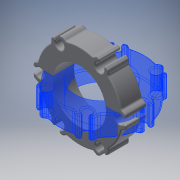
# Autodesk Inventor part: New Spacer
Saved by Autodesk Inventor 2017 (Build 210142000, 142)
## iProperties
Created: 2019-02-09
Part Number: New Spacer
Material: Generic
Document SubType Name: Modeling
Designer: S346795925
Density: 1 g/cm^3
Appearance: Default
Author: S346795925
Autodesk Inventor part; units mm, degrees
ref_plane "YZ Plane" through (0, 0, 0) normal (1, 0, 0) x (0, 1, 0)
ref_plane "XZ Plane" through (0, 0, 0) normal (0, 1, 0) x (-1, 0, 0)
ref_plane "XY Plane" through (0, 0, 0) normal (0, 0, 1) x (1, 0, 0)
sketch "Sketch1" plane through (0, 0, 0) normal (0, 0, 1) x (1, 0, 0)
  arc A0 (-16.7237, 21.3145) -> (-16.6929, 19.7418) centre (-11.9062, 20.6222) ccw construction
  arc A1 (-17.2068, 18.1665) -> (-16.6929, 19.7418) centre (-18.4013, 19.4276) ccw construction
  arc A2 (-17.2068, 18.1665) -> (-24.336, 5.8183) centre (0, 0) ccw construction
  arc A3 (-25.4434, 4.5856) -> (-24.336, 5.8183) centre (-26.0254, 6.2222) ccw construction
  arc A4 (-25.4434, 4.5856) -> (-26.8208, 3.8259) centre (-23.8125, 0) ccw construction
  arc A5 (-26.8208, 3.8259) -> (-27.1216, 3.2914) centre (-26.3245, 3.1947) ccw construction
  arc A6 (-27.1216, 3.2914) -> (-27.2147, 2.4031) centre (0, 0) ccw construction
  arc A7 (-27.2147, 2.4031) -> (-26.8956, 2.0545) centre (-26.8956, 2.3749) ccw construction
  line L0 (-26.8956, 2.0545) -> (-26.215, 2.0545) construction
  arc A8 (-26.215, 2.0545) -> (-25.9872, 2.1497) centre (-26.215, 2.3749) ccw construction
  arc A9 (-25.9872, -2.1497) -> (-25.9872, 2.1497) centre (-23.8125, 0) ccw construction
  arc A10 (-25.9872, -2.1497) -> (-26.215, -2.0545) centre (-26.215, -2.3749) ccw construction
  line L1 (-26.215, -2.0545) -> (-26.8956, -2.0545) construction
  arc A11 (-26.8956, -2.0545) -> (-27.2147, -2.4031) centre (-26.8956, -2.3749) ccw construction
  arc A12 (-27.2147, -2.4031) -> (-27.1216, -3.2914) centre (0, 0) ccw construction
  arc A13 (-27.1216, -3.2914) -> (-26.8208, -3.8259) centre (-26.3245, -3.1947) ccw construction
  arc A14 (-26.8208, -3.8259) -> (-24.5552, -4.81) centre (-23.8125, 0) ccw construction
  arc A15 (-24.5552, -4.81) -> (-17.2068, -18.1665) centre (0, 0) ccw construction
  arc A16 (-16.6929, -19.7418) -> (-17.2068, -18.1665) centre (-18.4013, -19.4276) ccw construction
  arc A17 (-16.6929, -19.7418) -> (-16.7237, -21.3145) centre (-11.9062, -20.6222) ccw construction
  arc A18 (-16.7237, -21.3145) -> (-16.4113, -21.8422) centre (-15.9289, -21.2003) ccw construction
  arc A19 (-16.4113, -21.8422) -> (-15.6885, -22.3671) centre (0, 0) ccw construction
  arc A20 (-15.6885, -22.3671) -> (-15.2271, -22.265) centre (-15.5045, -22.1048) ccw construction
  line L2 (-15.2271, -22.265) -> (-14.8868, -21.6756) construction
  arc A21 (-14.8868, -21.6756) -> (-14.8553, -21.4307) centre (-15.1642, -21.5154) ccw construction
  arc A22 (-11.1319, -23.5804) -> (-14.8553, -21.4307) centre (-11.9062, -20.6222) ccw construction
  arc A23 (-11.1319, -23.5804) -> (-11.3282, -23.7301) centre (-11.0508, -23.8903) ccw construction
  line L3 (-11.3282, -23.7301) -> (-11.6685, -24.3195) construction
  arc A24 (-11.6685, -24.3195) -> (-11.5262, -24.7701) centre (-11.3911, -24.4797) ccw construction
  arc A25 (-11.5262, -24.7701) -> (-10.7103, -25.1337) centre (0, 0) ccw construction
  arc A26 (-10.7103, -25.1337) -> (-10.097, -25.1404) centre (-10.3955, -24.395) ccw construction
  arc A27 (-10.097, -25.1404) -> (-8.7504, -24.3274) centre (-11.9062, -20.6222) ccw construction
  arc A28 (-7.1292, -23.9847) -> (-8.7504, -24.3274) centre (-7.6241, -25.6498) ccw construction
  arc A29 (-7.1292, -23.9847) -> (7.1292, -23.9847) centre (0, 0) ccw construction
  arc A30 (8.7504, -24.3274) -> (7.1292, -23.9847) centre (7.6241, -25.6498) ccw construction
  arc A31 (8.7504, -24.3274) -> (10.097, -25.1404) centre (11.9063, -20.6222) ccw construction
  arc A32 (10.097, -25.1404) -> (10.7103, -25.1337) centre (10.3955, -24.395) ccw construction
  arc A33 (10.7103, -25.1337) -> (11.5262, -24.7701) centre (0, 0) ccw construction
  arc A34 (11.5262, -24.7701) -> (11.6685, -24.3195) centre (11.3911, -24.4797) ccw construction
  line L4 (11.6685, -24.3195) -> (11.3282, -23.7301) construction
  arc A35 (11.3282, -23.7301) -> (11.1319, -23.5804) centre (11.0508, -23.8903) ccw construction
  arc A36 (14.8553, -21.4307) -> (11.1319, -23.5804) centre (11.9063, -20.6222) ccw construction
  arc A37 (14.8553, -21.4307) -> (14.8868, -21.6756) centre (15.1642, -21.5154) ccw construction
  line L5 (14.8868, -21.6756) -> (15.2271, -22.265) construction
  arc A38 (15.2271, -22.265) -> (15.6885, -22.3671) centre (15.5045, -22.1048) ccw construction
  arc A39 (15.6885, -22.3671) -> (16.4113, -21.8422) centre (0, 0) ccw construction
  arc A40 (16.4113, -21.8422) -> (16.7237, -21.3145) centre (15.9289, -21.2003) ccw construction
  arc A41 (16.7237, -21.3145) -> (16.6929, -19.7418) centre (11.9063, -20.6222) ccw construction
  arc A42 (17.2068, -18.1665) -> (16.6929, -19.7418) centre (18.4013, -19.4276) ccw construction
  arc A43 (17.2068, -18.1665) -> (24.336, -5.8183) centre (0, 0) ccw construction
  arc A44 (25.4434, -4.5856) -> (24.336, -5.8183) centre (26.0254, -6.2222) ccw construction
  arc A45 (25.4434, -4.5856) -> (26.8208, -3.8259) centre (23.8125, 0) ccw construction
  arc A46 (26.8208, -3.8259) -> (27.1216, -3.2914) centre (26.3245, -3.1947) ccw construction
  arc A47 (27.1216, -3.2914) -> (27.2147, -2.4031) centre (0, 0) ccw construction
  arc A48 (27.2147, -2.4031) -> (26.8956, -2.0545) centre (26.8956, -2.3749) ccw construction
  line L6 (26.8956, -2.0545) -> (26.215, -2.0545) construction
  arc A49 (26.215, -2.0545) -> (25.9872, -2.1497) centre (26.215, -2.3749) ccw construction
  arc A50 (25.9872, 2.1497) -> (25.9872, -2.1497) centre (23.8125, 0) ccw construction
  arc A51 (25.9872, 2.1497) -> (26.215, 2.0545) centre (26.215, 2.3749) ccw construction
  line L7 (26.215, 2.0545) -> (26.8956, 2.0545) construction
  arc A52 (26.8956, 2.0545) -> (27.2147, 2.4031) centre (26.8956, 2.3749) ccw construction
  arc A53 (27.2147, 2.4031) -> (27.1216, 3.2914) centre (0, 0) ccw construction
  arc A54 (27.1216, 3.2914) -> (26.8208, 3.8259) centre (26.3245, 3.1947) ccw construction
  arc A55 (26.8208, 3.8259) -> (25.4434, 4.5856) centre (23.8125, 0) ccw construction
  arc A56 (24.336, 5.8183) -> (25.4434, 4.5856) centre (26.0254, 6.2222) ccw construction
  arc A57 (24.336, 5.8183) -> (17.2068, 18.1665) centre (0, 0) ccw construction
  arc A58 (16.6929, 19.7418) -> (17.2068, 18.1665) centre (18.4013, 19.4276) ccw construction
  arc A59 (16.6929, 19.7418) -> (16.7237, 21.3145) centre (11.9063, 20.6222) ccw construction
  arc A60 (16.7237, 21.3145) -> (16.4113, 21.8422) centre (15.9289, 21.2003) ccw construction
  arc A61 (16.4113, 21.8422) -> (15.6885, 22.3671) centre (0, 0) ccw construction
  arc A62 (15.6885, 22.3671) -> (15.2271, 22.265) centre (15.5045, 22.1048) ccw construction
  line L8 (15.2271, 22.265) -> (14.8868, 21.6756) construction
  arc A63 (14.8868, 21.6756) -> (14.8553, 21.4307) centre (15.1642, 21.5154) ccw construction
  arc A64 (11.1319, 23.5804) -> (14.8553, 21.4307) centre (11.9063, 20.6222) ccw construction
  arc A65 (11.1319, 23.5804) -> (11.3282, 23.7301) centre (11.0508, 23.8903) ccw construction
  line L9 (11.3282, 23.7301) -> (11.6685, 24.3195) construction
  arc A66 (11.6685, 24.3195) -> (11.5262, 24.7701) centre (11.3911, 24.4797) ccw construction
  arc A67 (11.5262, 24.7701) -> (10.7103, 25.1337) centre (0, 0) ccw construction
  arc A68 (10.7103, 25.1337) -> (10.097, 25.1404) centre (10.3955, 24.395) ccw construction
  arc A69 (10.097, 25.1404) -> (8.7504, 24.3274) centre (11.9063, 20.6222) ccw construction
  arc A70 (7.1292, 23.9847) -> (8.7504, 24.3274) centre (7.6241, 25.6498) ccw construction
  arc A71 (7.1292, 23.9847) -> (-7.1292, 23.9847) centre (0, 0) ccw construction
  arc A72 (-8.7504, 24.3274) -> (-7.1292, 23.9847) centre (-7.6241, 25.6498) ccw construction
  arc A73 (-8.7504, 24.3274) -> (-10.097, 25.1404) centre (-11.9062, 20.6222) ccw construction
  arc A74 (-10.097, 25.1404) -> (-10.7103, 25.1337) centre (-10.3955, 24.395) ccw construction
  arc A75 (-10.7103, 25.1337) -> (-11.5262, 24.7701) centre (0, 0) ccw construction
  arc A76 (-11.5262, 24.7701) -> (-11.6685, 24.3195) centre (-11.3911, 24.4797) ccw construction
  line L10 (-11.6685, 24.3195) -> (-11.3282, 23.7301) construction
  arc A77 (-11.3282, 23.7301) -> (-11.1319, 23.5804) centre (-11.0508, 23.8903) ccw construction
  arc A78 (-14.8553, 21.4307) -> (-11.1319, 23.5804) centre (-11.9062, 20.6222) ccw construction
  arc A79 (-14.8553, 21.4307) -> (-14.8868, 21.6756) centre (-15.1642, 21.5154) ccw construction
  line L11 (-14.8868, 21.6756) -> (-15.2271, 22.265) construction
  arc A80 (-15.2271, 22.265) -> (-15.6885, 22.3671) centre (-15.5045, 22.1048) ccw construction
  arc A81 (-15.6885, 22.3671) -> (-16.4113, 21.8422) centre (0, 0) ccw construction
  arc A82 (-16.4113, 21.8422) -> (-16.7237, 21.3145) centre (-15.9289, 21.2003) ccw construction
  circle A83 centre (0, 0) radius 16.138 construction
  arc A84 (-24.9427, -5.2035) -> (-17.5216, -18.4989) centre (0, 0) ccw construction
  circle A85 centre (0, 0) radius 15.8842 projected
  arc A86 (-24.9427, -5.2035) -> (-17.5216, -18.4989) centre (0, 0) ccw
  arc A87 (-27.1038, -4.1858) -> (-24.9427, -5.2035) centre (-23.8125, 0) ccw
  arc A88 (-27.5761, -3.3466) -> (-27.1038, -4.1858) centre (-26.3245, -3.1947) ccw
  arc A89 (-27.6708, -2.4434) -> (-27.5761, -3.3466) centre (0, 0) ccw
  arc A90 (-26.8956, -1.5967) -> (-27.6708, -2.4434) centre (-26.8956, -2.3749) ccw
  line L12 (-26.8956, -1.5967) -> (-26.215, -1.5967)
  arc A91 (-25.6616, -1.8278) -> (-26.215, -1.5967) centre (-26.215, -2.3749) ccw
  arc A92 (-25.6616, -1.8278) -> (-25.6616, 1.8278) centre (-23.8125, 0) ccw
  arc A93 (-26.215, 1.5967) -> (-25.6616, 1.8278) centre (-26.215, 2.3749) ccw
  line L13 (-26.215, 1.5967) -> (-26.8956, 1.5967)
  arc A94 (-27.6708, 2.4434) -> (-26.8956, 1.5967) centre (-26.8956, 2.3749) ccw
  arc A95 (-27.5761, 3.3466) -> (-27.6708, 2.4434) centre (0, 0) ccw
  arc A96 (-27.1038, 4.1858) -> (-27.5761, 3.3466) centre (-26.3245, 3.1947) ccw
  arc A97 (-25.5968, 5.017) -> (-27.1038, 4.1858) centre (-23.8125, 0) ccw
  arc A98 (-25.5968, 5.017) -> (-24.7813, 5.9248) centre (-26.0254, 6.2222) ccw
  arc A99 (-17.5216, 18.4989) -> (-24.7813, 5.9248) centre (0, 0) ccw
  arc A100 (-17.5216, 18.4989) -> (-17.1432, 19.659) centre (-18.4013, 19.4276) ccw
  arc A101 (-17.1769, 21.3796) -> (-17.1432, 19.659) centre (-11.9062, 20.6222) ccw
  arc A102 (-16.6863, 22.2083) -> (-17.1769, 21.3796) centre (-15.9289, 21.2003) ccw
  arc A103 (-15.9514, 22.7419) -> (-16.6863, 22.2083) centre (0, 0) ccw
  arc A104 (-14.8305, 22.4939) -> (-15.9514, 22.7419) centre (-15.5045, 22.1048) ccw
  line L14 (-14.8305, 22.4939) -> (-14.4903, 21.9045)
  arc A105 (-14.4137, 21.3097) -> (-14.4903, 21.9045) centre (-15.1642, 21.5154) ccw
  arc A106 (-14.4137, 21.3097) -> (-11.2479, 23.1375) centre (-11.9062, 20.6222) ccw
  arc A107 (-11.7247, 23.5012) -> (-11.2479, 23.1375) centre (-11.0508, 23.8903) ccw
  line L15 (-11.7247, 23.5012) -> (-12.065, 24.0906)
  arc A108 (-11.7194, 25.1853) -> (-12.065, 24.0906) centre (-11.3911, 24.4797) ccw
  arc A109 (-10.8898, 25.5549) -> (-11.7194, 25.1853) centre (0, 0) ccw
  arc A110 (-9.9268, 25.5655) -> (-10.8898, 25.5549) centre (-10.3955, 24.395) ccw
  arc A111 (-8.4536, 24.676) -> (-9.9268, 25.5655) centre (-11.9062, 20.6222) ccw
  arc A112 (-8.4536, 24.676) -> (-7.2597, 24.4236) centre (-7.6241, 25.6498) ccw
  arc A113 (7.2597, 24.4236) -> (-7.2597, 24.4236) centre (0, 0) ccw
  arc A114 (7.2597, 24.4236) -> (8.4536, 24.676) centre (7.6241, 25.6498) ccw
  arc A115 (9.9268, 25.5655) -> (8.4536, 24.676) centre (11.9063, 20.6222) ccw
  arc A116 (10.8898, 25.5549) -> (9.9268, 25.5655) centre (10.3955, 24.395) ccw
  arc A117 (11.7194, 25.1853) -> (10.8898, 25.5549) centre (0, 0) ccw
  arc A118 (12.065, 24.0906) -> (11.7194, 25.1853) centre (11.3911, 24.4797) ccw
  line L16 (12.065, 24.0906) -> (11.7247, 23.5012)
  arc A119 (11.2479, 23.1375) -> (11.7247, 23.5012) centre (11.0508, 23.8903) ccw
  arc A120 (11.2479, 23.1375) -> (14.4137, 21.3097) centre (11.9063, 20.6222) ccw
  arc A121 (14.4903, 21.9045) -> (14.4137, 21.3097) centre (15.1642, 21.5154) ccw
  line L17 (14.4903, 21.9045) -> (14.8305, 22.4939)
  arc A122 (15.9514, 22.7419) -> (14.8305, 22.4939) centre (15.5045, 22.1048) ccw
  arc A123 (16.6863, 22.2083) -> (15.9514, 22.7419) centre (0, 0) ccw
  arc A124 (17.1769, 21.3796) -> (16.6863, 22.2083) centre (15.9289, 21.2003) ccw
  arc A125 (17.1432, 19.659) -> (17.1769, 21.3796) centre (11.9063, 20.6222) ccw
  arc A126 (17.1432, 19.659) -> (17.5216, 18.4989) centre (18.4013, 19.4276) ccw
  arc A127 (24.7813, 5.9248) -> (17.5216, 18.4989) centre (0, 0) ccw
  arc A128 (24.7813, 5.9248) -> (25.5968, 5.017) centre (26.0254, 6.2222) ccw
  arc A129 (27.1038, 4.1858) -> (25.5968, 5.017) centre (23.8125, 0) ccw
  arc A130 (27.5761, 3.3466) -> (27.1038, 4.1858) centre (26.3245, 3.1947) ccw
  arc A131 (27.6708, 2.4434) -> (27.5761, 3.3466) centre (0, 0) ccw
  arc A132 (26.8956, 1.5967) -> (27.6708, 2.4434) centre (26.8956, 2.3749) ccw
  line L18 (26.8956, 1.5967) -> (26.215, 1.5967)
  arc A133 (25.6616, 1.8278) -> (26.215, 1.5967) centre (26.215, 2.3749) ccw
  arc A134 (25.6616, 1.8278) -> (25.6616, -1.8278) centre (23.8125, 0) ccw
  arc A135 (26.215, -1.5967) -> (25.6616, -1.8278) centre (26.215, -2.3749) ccw
  line L19 (26.215, -1.5967) -> (26.8956, -1.5967)
  arc A136 (27.6708, -2.4434) -> (26.8956, -1.5967) centre (26.8956, -2.3749) ccw
  arc A137 (27.5761, -3.3466) -> (27.6708, -2.4434) centre (0, 0) ccw
  arc A138 (27.1038, -4.1858) -> (27.5761, -3.3466) centre (26.3245, -3.1947) ccw
  arc A139 (25.5968, -5.017) -> (27.1038, -4.1858) centre (23.8125, 0) ccw
  arc A140 (25.5968, -5.017) -> (24.7813, -5.9248) centre (26.0254, -6.2222) ccw
  arc A141 (17.5216, -18.4989) -> (24.7813, -5.9248) centre (0, 0) ccw
  arc A142 (17.5216, -18.4989) -> (17.1432, -19.659) centre (18.4013, -19.4276) ccw
  arc A143 (17.1769, -21.3796) -> (17.1432, -19.659) centre (11.9063, -20.6222) ccw
  arc A144 (16.6863, -22.2083) -> (17.1769, -21.3796) centre (15.9289, -21.2003) ccw
  arc A145 (15.9514, -22.7419) -> (16.6863, -22.2083) centre (0, 0) ccw
  arc A146 (14.8305, -22.4939) -> (15.9514, -22.7419) centre (15.5045, -22.1048) ccw
  line L20 (14.8305, -22.4939) -> (14.4903, -21.9045)
  arc A147 (14.4137, -21.3097) -> (14.4903, -21.9045) centre (15.1642, -21.5154) ccw
  arc A148 (14.4137, -21.3097) -> (11.2479, -23.1375) centre (11.9063, -20.6222) ccw
  arc A149 (11.7247, -23.5012) -> (11.2479, -23.1375) centre (11.0508, -23.8903) ccw
  line L21 (11.7247, -23.5012) -> (12.065, -24.0906)
  arc A150 (11.7194, -25.1853) -> (12.065, -24.0906) centre (11.3911, -24.4797) ccw
  arc A151 (10.8898, -25.5549) -> (11.7194, -25.1853) centre (0, 0) ccw
  arc A152 (9.9268, -25.5655) -> (10.8898, -25.5549) centre (10.3955, -24.395) ccw
  arc A153 (8.4536, -24.676) -> (9.9268, -25.5655) centre (11.9063, -20.6222) ccw
  arc A154 (8.4536, -24.676) -> (7.2597, -24.4236) centre (7.6241, -25.6498) ccw
  arc A155 (-7.2597, -24.4236) -> (7.2597, -24.4236) centre (0, 0) ccw
  arc A156 (-7.2597, -24.4236) -> (-8.4536, -24.676) centre (-7.6241, -25.6498) ccw
  arc A157 (-9.9268, -25.5655) -> (-8.4536, -24.676) centre (-11.9062, -20.6222) ccw
  arc A158 (-10.8898, -25.5549) -> (-9.9268, -25.5655) centre (-10.3955, -24.395) ccw
  arc A159 (-11.7194, -25.1853) -> (-10.8898, -25.5549) centre (0, 0) ccw
  arc A160 (-12.065, -24.0906) -> (-11.7194, -25.1853) centre (-11.3911, -24.4797) ccw
  line L22 (-12.065, -24.0906) -> (-11.7247, -23.5012)
  arc A161 (-11.2479, -23.1375) -> (-11.7247, -23.5012) centre (-11.0508, -23.8903) ccw
  arc A162 (-11.2479, -23.1375) -> (-14.4137, -21.3097) centre (-11.9062, -20.6222) ccw
  arc A163 (-14.4903, -21.9045) -> (-14.4137, -21.3097) centre (-15.1642, -21.5154) ccw
  line L23 (-14.4903, -21.9045) -> (-14.8305, -22.4939)
  arc A164 (-15.9514, -22.7419) -> (-14.8305, -22.4939) centre (-15.5045, -22.1048) ccw
  arc A165 (-16.6863, -22.2083) -> (-15.9514, -22.7419) centre (0, 0) ccw
  arc A166 (-17.1769, -21.3796) -> (-16.6863, -22.2083) centre (-15.9289, -21.2003) ccw
  arc A167 (-17.1432, -19.659) -> (-17.1769, -21.3796) centre (-11.9062, -20.6222) ccw
  arc A168 (-17.1432, -19.659) -> (-17.5216, -18.4989) centre (-18.4013, -19.4276) ccw
  constraints: 166 point on circle, 83 centre point, 24 end point, 94 other
extrude "Extrusion1" add sketch "Sketch1" along normal blind 12.7
fillet "Fillet1" radius 0.762 190 edges at (17.1852, 19.0309, 12.7) (17.23, 20.5179, 12.7) (17.0138, 21.8426, 12.7) (16.321, 22.4781, 12.7) (15.3364, 22.8646, 12.7) (14.6604, 22.1992, 12.7) (14.3924, 21.6148, 12.7) (10.6063, 18.3706, 12.7) (11.5227, 23.2715, 12.7) (11.8949, 23.7959, 12.7) (12.1332, 24.714, 12.7) (11.3061, 25.3735, 12.7) (10.4094, 25.6557, 12.7) (9.154, 25.1806, 12.7) (7.8886, 24.3983, 12.7) (0, 25.4797, 12.7) (-7.8886, 24.3983, 12.7) (-9.154, 25.1806, 12.7) (-10.4094, 25.6557, 12.7) (-11.3061, 25.3735, 12.7) (-12.1332, 24.714, 12.7) (-11.8949, 23.7959, 12.7) (-11.5227, 23.2715, 12.7) (-10.6063, 18.3706, 12.7) (-14.3924, 21.6148, 12.7) (-14.6604, 22.1992, 12.7) (-15.3364, 22.8646, 12.7) (-16.321, 22.4781, 12.7) (-17.0138, 21.8426, 12.7) (-17.23, 20.5179, 12.7) (-17.1852, 19.0309, 12.7) (-22.0661, 12.7399, 12.7) (-25.0738, 5.3674, 12.7) (-26.3841, 4.6627, 12.7) (-27.4232, 3.8131, 12.7) (-27.6271, 2.8954, 12.7) (-27.4695, 1.8494, 12.7) (-26.5553, 1.5967, 12.7) (-25.9151, 1.6568, 12.7) (-21.2125, 0, 12.7) (-25.9151, -1.6568, 12.7) (-26.5553, -1.5967, 12.7) (-27.4695, -1.8494, 12.7) (-27.6271, -2.8954, 12.7) (-27.4232, -3.8131, 12.7) (-26.081, -4.8174, 12.7) (25.0738, 5.3674, 12.7) (26.3841, 4.6627, 12.7) (27.4232, 3.8131, 12.7) (27.6271, 2.8954, 12.7) (27.4695, 1.8494, 12.7) (26.5553, 1.5967, 12.7) (25.9151, 1.6568, 12.7) (21.2125, 0, 12.7) (25.9151, -1.6568, 12.7) (26.5553, -1.5967, 12.7) (27.4695, -1.8494, 12.7) (27.6271, -2.8954, 12.7) (27.4232, -3.8131, 12.7) (26.3841, -4.6627, 12.7) (25.0738, -5.3674, 12.7) (22.0661, -12.7399, 12.7) (17.1852, -19.0309, 12.7) (17.23, -20.5179, 12.7) (17.0138, -21.8426, 12.7) (16.321, -22.4781, 12.7) (15.3364, -22.8646, 12.7) (14.6604, -22.1992, 12.7) (14.3924, -21.6148, 12.7) (10.6063, -18.3706, 12.7) (11.5227, -23.2715, 12.7) (11.8949, -23.7959, 12.7) (12.1332, -24.714, 12.7) (11.3061, -25.3735, 12.7) (10.4094, -25.6557, 12.7) (9.154, -25.1806, 12.7) (7.8886, -24.3983, 12.7) (0, -25.4797, 12.7) (-7.8886, -24.3983, 12.7) (-9.154, -25.1806, 12.7) (-10.4094, -25.6557, 12.7) (-11.3061, -25.3735, 12.7) (-12.1332, -24.714, 12.7) (-11.8949, -23.7959, 12.7) (-11.5227, -23.2715, 12.7) (-10.6063, -18.3706, 12.7) (-14.3924, -21.6148, 12.7) (-14.6604, -22.1992, 12.7) (-15.3364, -22.8646, 12.7) (-16.321, -22.4781, 12.7) (-17.0138, -21.8426, 12.7) (-17.23, -20.5179, 12.7) (-17.1852, -19.0309, 12.7) (-22.2485, -12.4185, 12.7) (22.0661, 12.7399, 12.7) (17.1852, 19.0309, 0) (17.23, 20.5179, 0) (17.0138, 21.8426, 0) (16.321, 22.4781, 0) (15.3364, 22.8646, 0) (14.6604, 22.1992, 0) (14.3924, 21.6148, 0) (10.6063, 18.3706, 0) (11.5227, 23.2715, 0) (11.8949, 23.7959, 0) (12.1332, 24.714, 0) (11.3061, 25.3735, 0) (10.4094, 25.6557, 0) (9.154, 25.1806, 0) (7.8886, 24.3983, 0) (0, 25.4797, 0) (-7.8886, 24.3983, 0) (-9.154, 25.1806, 0) (-10.4094, 25.6557, 0) (-11.3061, 25.3735, 0) (-12.1332, 24.714, 0) (-11.8949, 23.7959, 0) (-11.5227, 23.2715, 0) (-10.6063, 18.3706, 0) (-14.3924, 21.6148, 0) (-14.6604, 22.1992, 0) (-15.3364, 22.8646, 0) (-16.321, 22.4781, 0) (-17.0138, 21.8426, 0) (-17.23, 20.5179, 0) (-17.1852, 19.0309, 0) (-22.0661, 12.7399, 0) (-25.0738, 5.3674, 0) (-26.3841, 4.6627, 0) (-27.4232, 3.8131, 0) (-27.6271, 2.8954, 0) (-27.4695, 1.8494, 0) (-26.5553, 1.5967, 0) (-25.9151, 1.6568, 0) (-21.2125, 0, 0) (-25.9151, -1.6568, 0) (-26.5553, -1.5967, 0) (-27.4695, -1.8494, 0) (-27.6271, -2.8954, 0) (-27.4232, -3.8131, 0) (-26.081, -4.8174, 0) (25.0738, 5.3674, 0) (26.3841, 4.6627, 0) (27.4232, 3.8131, 0) (27.6271, 2.8954, 0) (27.4695, 1.8494, 0) (26.5553, 1.5967, 0) (25.9151, 1.6568, 0) (21.2125, 0, 0) (25.9151, -1.6568, 0) (26.5553, -1.5967, 0) (27.4695, -1.8494, 0) (27.6271, -2.8954, 0) (27.4232, -3.8131, 0) (26.3841, -4.6627, 0) (25.0738, -5.3674, 0) (22.0661, -12.7399, 0) (17.1852, -19.0309, 0) (17.23, -20.5179, 0) (17.0138, -21.8426, 0) (16.321, -22.4781, 0) (15.3364, -22.8646, 0) (14.6604, -22.1992, 0) (14.3924, -21.6148, 0) (10.6063, -18.3706, 0) (11.5227, -23.2715, 0) (11.8949, -23.7959, 0) (12.1332, -24.714, 0) (11.3061, -25.3735, 0) (10.4094, -25.6557, 0) (9.154, -25.1806, 0) (7.8886, -24.3983, 0) (0, -25.4797, 0) (-7.8886, -24.3983, 0) (-9.154, -25.1806, 0) (-10.4094, -25.6557, 0) (-11.3061, -25.3735, 0) (-12.1332, -24.714, 0) (-11.8949, -23.7959, 0) (-11.5227, -23.2715, 0) (-10.6063, -18.3706, 0) (-14.3924, -21.6148, 0) (-14.6604, -22.1992, 0) (-15.3364, -22.8646, 0) (-16.321, -22.4781, 0) (-17.0138, -21.8426, 0) (-17.23, -20.5179, 0) (-17.1852, -19.0309, 0) (-22.2485, -12.4185, 0) (22.0661, 12.7399, 0)
body "Solid1"
